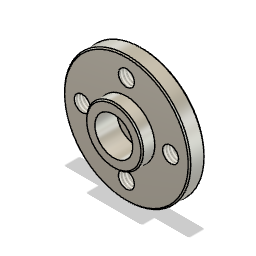
GooGoo (Autodesk Fusion 360 archive; units mm, degrees)
design "Servo Disc"
Autodesk Fusion 360 part; units mm, degrees
note: some values were not read from the file. Set by a fixed rule: which face or edge a step refers to.
sketch "Sketch1" plane through (0, 0, 0) normal (0, 0, 1) x (1, 0, 0)
  circle A0 centre (0, 0) radius 10
  dimension "d1" = 20
  constraint coincident A0.centre origin
  measures "d1" diameter of A0
extrude "Extrude1" add sketch "Sketch1" along normal blind 2.5
sketch "Sketch2" plane through (0, 0, 2.5) normal (0, 0, 1) x (1, 0, 0)
  circle A0 centre (0, 0) radius 10
  circle A1 centre (0, 0) radius 4.5
  dimension "d4" = 9
  constraint concentric A0 A1
  measures "d4" diameter of A1
extrude "Extrude2" add sketch "Sketch2" along normal blind 2 contours A1
sketch "Sketch3" plane through (0, 0, 2.5) normal (0, 0, 1) x (1, 0, 0)
  circle A0 centre (0, 0) radius 4.5
  circle A1 centre (0, 0) radius 10
  line L0 (0, 0) -> (0, 7)
  point P0 (0, 7)
  dimension "d8" = 7
  constraint coincident A0.centre A1.centre
  constraint vertical L0
  constraint coincident P0 L0.end
  measures "d8" distance of A0.centre P0
hole "Hole1" at (0, 7, 2.5) direction (0, 0, -1) diameter 2.529 depth 9 tip angle 118
thread "Thread1" "ISO Metric profile 3.0 M3x0.5 6H"
pattern_circular "C-Pattern1" count 4 over 360 about axis through (0, 0, 0) along (0, 0, 1) of "Hole1"
sketch "Sketch4" plane through (0, 0, 4.5) normal (0, 0, 1) x (1, 0, 0)
  circle A0 centre (0, 0) radius 3
  circle A1 centre (0, 0) radius 4.5
  dimension "d14" = 6
  measures "d14" diameter of A0
extrude "Extrude3" cut sketch "Sketch4" against normal blind 3.5 contours A0
sketch "Sketch5" plane through (0, 0, 1) normal (0, 0, 1) x (1, 0, 0)
  circle A0 centre (0, 0) radius 3
  circle A1 centre (0, 0) radius 1.5
  dimension "d17" = 3
  constraint coincident A0.centre A1.centre
  measures "d17" diameter of A1
extrude "Extrude4" cut sketch "Sketch5" against normal blind 3 contours A1
chamfer "Chamfer1" distance 0.2 angle 45 4 edges at (-4.1955, -1.6273, 4.5) (-9.3233, -3.6162, 2.5) (-9.3233, -3.6162, 0) (-1.3985, -0.5424, 0)

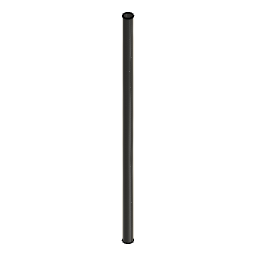
design "20x18x500CR"
Autodesk Fusion 360 part; units mm, degrees
sketch "Sketch1" plane through (0, 0, 0) normal (0, 0, 1) x (1, 0, 0)
  circle A0 centre (0, 0) radius 10
  circle A1 centre (0, 0) radius 9
  dimension "d1" = 20
  dimension "d2" = 18
  constraint coincident A0.centre A1.centre
  measures "d1" diameter of A0
  measures "d2" diameter of A1
extrude "Extrude1" add sketch "Sketch1" along normal blind 500

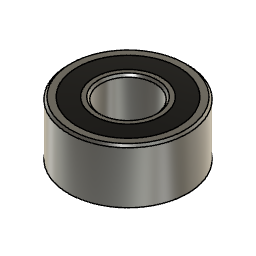
design "5x11x5mmBearing"
Autodesk Fusion 360 part; units mm, degrees
sketch "Sketch1" plane through (0, 0, 0) normal (0, 0, 1) x (1, 0, 0)
  circle A0 centre (0, 0) radius 2.5
  circle A1 centre (0, 0) radius 3.1
  circle A2 centre (0, 0) radius 5.5
  circle A3 centre (0, 0) radius 4.7
  dimension "d1" = 5
  dimension "d2" = 0.6
  dimension "d3" = 11
  dimension "d4" = -0.8
  constraint coincident A0.centre A1.centre
  measures "d1" diameter of A0
  measures "d3" diameter of A2
extrude "Extrude1" add sketch "Sketch1" along normal blind 5 makes body 1 at (5.4932, -0.2742, 3.3333) makes body 2 at (3.0961, -0.1545, 3.3333)
extrude "Extrude2" add sketch "Sketch1" along normal blind 5 separate body contours A3 makes body 3
chamfer "Chamfer1" distance 0.2 angle 45 2 edges at (-5.1278, -1.9889, 5) (-2.3308, 0.904, 5) on bodies 1 2

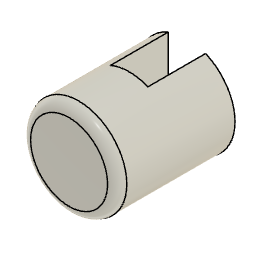
design "PegCR"
Autodesk Fusion 360 part; units mm, degrees
sketch "Sketch1" plane through (0, 0, 0) normal (0, 1, 0) x (1, 0, 0)
  circle A0 centre (0, 0) radius 4
  line L0 (1.55, -6.2) -> (-1.55, -6.2)
  line L1 (-1.55, -6.2) -> (-1.55, 6.2)
  line L2 (-1.55, 6.2) -> (1.55, 6.2)
  line L3 (1.55, 6.2) -> (1.55, -6.2)
  line L4 (1.55, -6.2) -> (-1.55, 6.2) construction
  line L5 (-1.55, -6.2) -> (1.55, 6.2) construction
  dimension "d1" = 8
  dimension "d2" = 3.1
  constraint coincident A0.centre origin
  constraint horizontal L0
  constraint perpendicular L0 L1
  constraint parallel L0 L2
  constraint parallel L1 L3
  constraint coincident L4 A0.centre
  constraint coincident L5 A0.centre
  measures "d1" diameter of A0
  measures "d2" distance of L1.end L2.end
extrude "Extrude1" add sketch "Sketch1" against normal blind 5 contours A0 L3 | A0 L1 L3 | A0 L1
extrude "Extrude2" add sketch "Sketch1" along normal blind 4.8 contours A0 L3 | A0 L1
fillet "Fillet1" radius 0.8 1 edges at (-3.7293, -5, -1.4465)

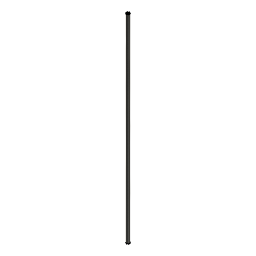
design "8x4x500CR"
Autodesk Fusion 360 part; units mm, degrees
sketch "Sketch1" plane through (0, 0, 0) normal (0, 0, 1) x (1, 0, 0)
  circle A0 centre (0, 0) radius 4
  circle A1 centre (0, 0) radius 2
  dimension "d1" = 8
  dimension "d2" = 4
  constraint coincident A0.centre A1.centre
  measures "d1" diameter of A0
  measures "d2" diameter of A1
extrude "Extrude1" add sketch "Sketch1" along normal blind 500

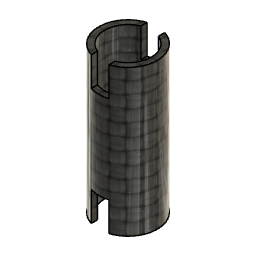
design "10x8x25CR"
Autodesk Fusion 360 part; units mm, degrees
sketch "Sketch1" plane through (0, 0, 0) normal (0, 0, 1) x (1, 0, 0)
  circle A0 centre (0, 0) radius 5
  circle A1 centre (0, 0) radius 4
  line L0 (1.5, 6) -> (-1.5, 6)
  line L1 (-1.5, 6) -> (-1.5, -6)
  line L2 (-1.5, -6) -> (1.5, -6)
  line L3 (1.5, -6) -> (1.5, 6)
  line L4 (1.5, 6) -> (-1.5, -6) construction
  line L5 (-1.5, 6) -> (1.5, -6) construction
  dimension "d1" = 10
  dimension "d2" = 8
  dimension "d3" = 3
  dimension "d4" = 12
  constraint coincident A0.centre A1.centre
  constraint horizontal L0
  constraint perpendicular L0 L1
  constraint parallel L0 L2
  constraint parallel L1 L3
  constraint coincident L4 A0.centre
  constraint coincident L5 A0.centre
  measures "d1" diameter of A0
  measures "d2" diameter of A1
  measures "d3" distance of L1.end L2.end
  measures "d4" distance of L0.end L1.end
extrude "Extrude1" add sketch "Sketch1" along normal blind 25 contours A0 A1 L3 | A0 A1 L1 L3 | A0 A1 L1 L3 | A0 A1 L1
sketch "Sketch2" plane through (0, 0, 25) normal (0, 0, 1) x (-1, 0, 0)
  circle A0 centre (0, 0) radius 4
  circle A1 centre (0, 0) radius 5
  line L0 (-1.5, -6) -> (1.5, -6)
  line L1 (1.5, -6) -> (1.5, 6)
  line L2 (1.5, 6) -> (-1.5, 6)
  line L3 (-1.5, 6) -> (-1.5, -6)
  line L4 (-1.5, -6) -> (1.5, 6) construction
  line L5 (1.5, -6) -> (-1.5, 6) construction
  dimension "d7" = 3
  dimension "d8" = 12
  constraint horizontal L0
  constraint perpendicular L0 L1
  constraint parallel L0 L2
  constraint parallel L1 L3
  constraint coincident L4 A0.centre
  constraint coincident L5 A0.centre
  constraint coincident A0.centre A1.centre
  measures "d7" distance of L1.end L2.end
  measures "d8" distance of L0.end L1.end
extrude "Extrude2" cut sketch "Sketch2" against normal blind 5 contours A0 A1 L1 L3 | A0 A1 L1 L3
extrude "Extrude3" cut sketch "Sketch1" along normal blind 5 contours A0 A1 L1 L3 | A0 A1 L1 L3

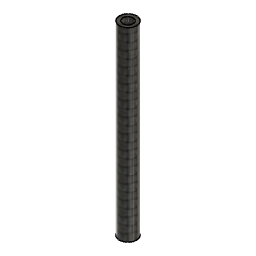
design "5x3x54CR"
Autodesk Fusion 360 part; units mm, degrees
sketch "Sketch1" plane through (0, 0, 0) normal (0, 0, 1) x (1, 0, 0)
  circle A0 centre (0, 0) radius 2.5
  circle A1 centre (0, 0) radius 1.5
  dimension "d1" = 5
  dimension "d2" = 3
  constraint coincident A0.centre A1.centre
  constraint concentric A0 A1
  measures "d1" diameter of A0
  measures "d2" diameter of A1
extrude "Extrude1" add sketch "Sketch1" along normal blind 54

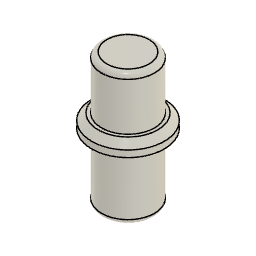
design "BearingCoupler"
Autodesk Fusion 360 part; units mm, degrees
sketch "Sketch1" plane through (0, 0, 0) normal (0, 0, 1) x (1, 0, 0)
  circle A0 centre (0, 0) radius 4
  circle A1 centre (0, 0) radius 5.5
  dimension "d1" = 8
  dimension "d13" = 11
  constraint coincident A0.centre A1.centre
  measures "d1" diameter of A0
  measures "d13" diameter of A1
extrude "Extrude1" add sketch "Sketch1" along normal blind 8 contours A0 makes body 1
extrude "Extrude2" add sketch "Sketch1" against normal blind 2 separate body makes body 2
extrude "Extrude3" add sketch "Sketch1" against normal blind 12 contours A0 bodies 1 2
fillet "Fillet1" radius 0.8 2 edges at (-3.7293, 1.4465, -12) (-3.7293, -1.4465, 8) on bodies 1
chamfer "Chamfer1" distance 1 angle 45 1 edges at (-5.1278, -1.9889, 0) on bodies 1

design "PropStructMount2"
Autodesk Fusion 360 part; units mm, degrees
sketch "Sketch1" plane through (0, 0, 0) normal (0, 1, 0) x (1, 0, 0)
  line L0 (0, 0) -> (-48, 0) construction
  line L1 (-48, 0) -> (-48, -15) construction
  line L2 (-48, -15) -> (-80, -15) construction
  line L3 (0, 0) -> (0, -70) construction
  circle A0 centre (0, -70) radius 10
  circle A1 centre (-80, -15) radius 4
  circle A2 centre (0, -70) radius 14
  circle A3 centre (-80, -15) radius 8
  line L4 (-84.931, -21.2996) -> (-8.6292, -81.0243)
  line L5 (-82.4655, -18.1498) -> (-6.1637, -77.8745)
  line L6 (0, -84) -> (0, -56)
  circle A4 centre (-48, 0) radius 11
  circle A5 centre (-48, 0) radius 15
  line L7 (0, -56) -> (-34.8639, 7.2417)
  line L8 (-2.6272, -57.4483) -> (-37.4911, 5.7933)
  line L9 (-84.7629, -8.5724) -> (-56.9305, 12.0518)
  line L10 (-82.3815, -11.7862) -> (-54.5491, 8.838)
  line L11 (-48, 15) -> (0, 15)
  line L12 (0, 15) -> (0, -56)
  dimension "d1" = 48
  dimension "d2" = 15
  dimension "d3" = 32
  dimension "d4" = 70
  dimension "d5" = 20
  dimension "d6" = 8
  dimension "d7" = 4
  dimension "d8" = 4
  dimension "d9" = 22
  dimension "d10" = 4
  dimension "d11" = -3
  dimension "d12" = 48
  constraint coincident L0.start L3.start
  constraint horizontal L0
  constraint perpendicular L0 L1
  constraint perpendicular L1 L2
  constraint perpendicular L0 L3
  constraint coincident L3.end A0.centre
  constraint coincident L2.end A1.centre
  constraint coincident A3 L4.start
  constraint coincident A2 L4.end
  constraint tangent A2 L4
  constraint coincident A1 L5.start
  constraint coincident A0 L5.end
  constraint tangent A0 L5
  constraint tangent A3 L4
  constraint tangent A1 L5
  constraint coincident A2 L6.start
  constraint coincident L3 L6.end
  constraint coincident A2 L6.end
  constraint parallel L3 L6
  constraint coincident L0.end L1.start
  constraint coincident A5 L7.end
  constraint tangent A5 L7
  constraint coincident A3 L9.start
  constraint coincident A5 L9.end
  constraint coincident A1 L10.start
  constraint coincident A4 L10.end
  constraint tangent A4 L10
  constraint tangent A5 L9
  constraint tangent A3 L9
  constraint tangent A1 L10
  constraint coincident A5 L11.start
  constraint parallel L0 L11
  constraint perpendicular L11 L12
  measures "d1" distance of L0.start L0.end
  measures "d2" distance of L0.end L1.end
  measures "d3" distance of L1.end L2.end
  measures "d4" distance of L0.start L3.end
  measures "d5" diameter of A0
  measures "d6" diameter of A1
  measures "d8" distance of A1
  measures "d9" diameter of A4
  measures "d12" distance of L11.start L11.end
extrude "Extrude1" add sketch "Sketch1" along normal blind 10 contours A0 A2 L5 L6 | A0 A2 L5 L6 | A2 A5 L7 L8 | A5 L7 L11 L12 | A2 A3 L5 A5 L8 L10 | A2 A3 L4 L5 | A5 | A1 A3 L5 L10 | A1 A3 L5 L10 | A3 A5 L9 L10
sketch "Sketch2" plane through (0, 0, 0) normal (0, -1, 0) x (1, 0, 0)
  circle A0 centre (-48, 0) radius 11
  circle A1 centre (-80, 15) radius 4
  arc A2 (-56.9305, -12.0518) -> (-48, -15) centre (-48, 0) ccw
  line L0 (-48, -15) -> (0, -15)
  line L1 (0, -15) -> (0, 60)
  arc A3 (0, 80) -> (0, 60) centre (0, 70) ccw
  line L2 (0, 80) -> (0, 84)
  arc A4 (0, 84) -> (-8.6292, 81.0243) centre (0, 70) ccw
  line L3 (-8.6292, 81.0243) -> (-84.931, 21.2996)
  arc A5 (-84.931, 21.2996) -> (-84.7629, 8.5724) centre (-80, 15) ccw
  line L4 (-84.7629, 8.5724) -> (-56.9305, -12.0518)
  circle A6 centre (-48, 0) radius 15
  circle A7 centre (-80, 15) radius 8
  circle A8 centre (0, 70) radius 14
  line L5 (-78.1065, 22.7727) -> (-44.4498, 14.5738)
  line L6 (-82.4655, 18.1498) -> (-6.1637, 77.8745)
  line L7 (0, 56) -> (-34.8639, -7.2417)
  circle A9 centre (0, 70) radius 10
  line L8 (-78.8166, 19.8579) -> (-45.1598, 11.659)
  line L9 (-82.3815, 11.7862) -> (-54.5491, -8.838)
  line L10 (-3.503, 57.9311) -> (-38.3668, -5.3106)
  line L11 (-13.8792, 71.8353) -> (-33.4434, 3.6203)
  line L12 (-16.7629, 72.6624) -> (-36.3272, 4.4473)
  circle A10 centre (0, -15) radius 34.2773
  circle A11 centre (0, -15) radius 38.2773
  dimension "d17" = 3
  dimension "d18" = -4
  dimension "d19" = 4
  dimension "d21" = 3
  dimension "d22" = 4
  constraint concentric A0 A6
  constraint concentric A1 A7
  constraint concentric A3 A8
  constraint coincident L2.end A8
  constraint coincident A7 L5.start
  constraint coincident A6 L5.end
  constraint tangent A6 L5
  constraint tangent A7 L5
  constraint coincident A1 L6.start
  constraint coincident A3 L6.end
  constraint tangent A3 L6
  constraint tangent A1 L6
  constraint coincident A8 L7.start
  constraint coincident L1 L7.start
  constraint coincident A6 L7.end
  constraint tangent A6 L7
  constraint concentric A8 A9
  constraint coincident L1.end A9
  constraint coincident A8 L11.start
  constraint coincident L6 L11.start
  constraint coincident A6 L11.end
  constraint coincident L10 L11.end
  constraint coincident L0.end L1.start
  constraint tangent L7 A10
extrude "Extrude2" cut sketch "Sketch2" against normal through all contours A8 L10 L11 | A6 A7 L8 L9 | A6 L5 L6 L12 | L1 L7 A11 | L0 A6 A11 | L0 A6 L7 A10 A11 | L0 L1 A10 picked at (-19.1897, -2.6862)
fillet "Fillet1" radius 1.5 2 edges at (-13.8792, 5, 71.8353) (-33.4434, 5, 3.6203)
fillet "Fillet2" radius 2 2 edges at (-17.9036, 5, 68.6853) (-76.9267, 5, 22.4853)
fillet "Fillet3" radius 2 1 edges at (-35.3093, 5, 7.9966)
fillet "Fillet4" radius 2 4 edges at (-53.9041, 5, 13.7892) (-72.749, 5, 18.3799) (-76.815, 5, 7.6614) (-62.7427, 5, -2.7664)
mirror "Mirror1" about plane through (0, 0, 0) normal (1, 0, 0) of bodies 1 merged
fillet "Fillet5" radius 1.2 2 edges at (-21.7936, 5, 16.4673) (21.7936, 5, 16.4673)
fillet "Fillet6" radius 3 3 edges at (-4.2103, 5, 56.6481) (0, 5, 56) (4.2103, 5, 56.6481)
ref_plane "WorkPlane1" through (0, 7, 0) normal (0, 1, 0) x (0, 0, 1)
sketch "Sketch3" plane through (0, 7, 0) normal (0, 1, 0) x (1, 0, 0)
  line L0 (0, 0) -> (48, 0) construction
  circle A0 centre (48, 0) radius 11.5
  circle A1 centre (48, 0) radius 7
  line L1 (0, 0) -> (0, -5) construction
  circle A2 centre (-48, 0) radius 7
  circle A3 centre (-48, 0) radius 11.5
  dimension "d36" = 48
  dimension "d37" = 23
  dimension "d38" = 14
  dimension "d39" = 5
  constraint coincident L0.start L1.start
  constraint horizontal L0
  constraint coincident L0.end A0.centre
  constraint concentric A0 A1
  constraint perpendicular L0 L1
  constraint symmetric A0 L1 A3
  constraint symmetric A1 L1 A2
  measures "d36" distance of L0.start L0.end
  measures "d37" diameter of A0
  measures "d38" diameter of A1
  measures "d39" distance of L0.start L1.end
extrude "Extrude3" add sketch "Sketch3" along normal blind 3
fillet "Fillet7" radius 1.5 48 faces at (19.0968, 3.3333, 18.765) (8.2897, 3.3333, 40.9627) (0, 3.3333, 52.786) (-8.2897, 3.3333, 40.9627) (-19.6699, 3.3333, 19.3747) (-11.4237, 6.6667, 21.5329) (20.521, 3.3333, 48.6773) (28.8377, 3.3333, 14.5841) (12.8668, 3.3333, 40.9455) (5.4179, 3.3333, 55.2754) (10.3943, 6.6667, 60.6213) (13.7109, 3.3333, 65.7014) (-12.8668, 6.6667, 40.9455) (-5.4179, 3.3333, 55.2754) (-10.3943, 6.6667, 60.6213) (-13.7109, 3.3333, 65.7014) (-20.521, 3.3333, 48.6773) (-28.8377, 3.3333, 14.5841) (63.4298, 3.3333, 19.1974) (73.7897, 6.6667, 21.9706) (56.7056, 3.3333, 38.3132) (22.5975, 3.3333, 64.9988) (24.4878, 3.3333, 45.7279) (37.4225, 6.6667, 10.6509) (38.056, 3.3333, 11.2302) (-63.4298, 3.3333, 19.1974) (-73.7897, 6.6667, 21.9706) (-56.7056, 6.6667, 38.3132) (-22.5975, 3.3333, 64.9988) (-24.4878, 3.3333, 45.7279) (-37.4225, 6.6667, 10.6509) (-38.056, 3.3333, 11.2302) (-61.0351, 6.6667, 7.4219) (-64.8968, 3.3333, -0.6439) (-71.7184, 6.6667, 3.8847) (-75.1274, 3.3333, 6.7064) (-72.0454, 6.6667, 14.1488) (-71.4826, 6.6667, 17.0228) (-65.8711, 3.3333, 16.7044) (-58.3295, 3.3333, 14.8574) (71.7184, 6.6667, 3.8847) (64.8968, 3.3333, -0.6439) (61.0351, 6.6667, 7.4219) (58.3295, 3.3333, 14.8574) (65.8711, 3.3333, 16.7044) (71.4826, 6.6667, 17.0228) (72.0454, 6.6667, 14.1488) (75.1274, 3.3333, 6.7064)
fillet "Fillet8" radius 1 24 edges at (46.7801, 0, 51.162) (87.9993, 0, 14.8944) (70.8467, 0, -1.7397) (44.8053, 0, -14.6559) (32.4409, 0, -2.8465) (0, 0, 19.2773) (-32.4409, 0, -2.8465) (-44.8053, 0, -14.6559) (-70.8467, 0, -1.7397) (-87.9993, 0, 14.8944) (-46.7801, 0, 51.162) (0, 0, 84) (46.7801, 10, 51.162) (87.9993, 10, 14.8944) (70.8467, 10, -1.7397) (44.8053, 10, -14.6559) (32.4409, 10, -2.8465) (0, 10, 19.2773) (-32.4409, 10, -2.8465) (-44.8053, 10, -14.6559) (-70.8467, 10, -1.7397) (-87.9993, 10, 14.8944) (-46.7801, 10, 51.162) (0, 10, 84)
sketch "Sketch5" plane through (0, 0, 0) normal (0, -1, 0) x (1, 0, 0)
  arc A0 (-69.1932, 19.0575) -> (-73.514, 15.427) centre (-70.0216, 15.657) ccw
  line L0 (-69.1932, 19.0575) -> (-73.2748, 20.0518)
  arc A1 (-74.6037, 26.2084) -> (-73.2748, 20.0518) centre (-72.4464, 23.4524) ccw
  line L1 (-74.6037, 26.2084) -> (-23.6831, 66.0662)
  arc A2 (-18.1614, 62.3452) -> (-23.6831, 66.0662) centre (-21.5258, 63.3101) ccw
  line L2 (-18.1614, 62.3452) -> (-17.3357, 65.2243)
  arc A3 (-11.6548, 65.4817) -> (-17.3357, 65.2243) centre (-14.452, 64.3973) ccw
  arc A4 (-11.6548, 65.4817) -> (-6.1894, 59.1399) centre (0, 70) ccw
  arc A5 (-4.4767, 53.0578) -> (-6.1894, 59.1399) centre (-8.4176, 55.2303) ccw
  line L3 (-4.4767, 53.0578) -> (-25.7061, 14.5485)
  arc A6 (-31.2171, 16.8239) -> (-25.7061, 14.5485) centre (-28.3333, 15.9968) ccw
  line L4 (-31.2171, 16.8239) -> (-32.8149, 11.2527)
  arc A7 (-38.613, 9.7022) -> (-32.8149, 11.2527) centre (-36.1793, 12.2176) ccw
  arc A8 (-38.613, 9.7022) -> (-44.8048, 13.1164) centre (-48, 0) ccw
  line L5 (-44.8048, 13.1164) -> (-58.1619, 16.3703)
  arc A9 (-56.7276, 10.2995) -> (-58.1619, 16.3703) centre (-58.9903, 12.9697) ccw
  arc A10 (-56.7276, 10.2995) -> (-61.457, 1.0764) centre (-48, 0) ccw
  arc A11 (-67.0297, -1.4566) -> (-61.457, 1.0764) centre (-64.9459, 1.3555) ccw
  line L6 (-67.0297, -1.4566) -> (-75.4023, 4.7476)
  arc A12 (-75.6571, 10.1638) -> (-75.4023, 4.7476) centre (-73.3185, 7.5597) ccw
  arc A13 (-75.6571, 10.1638) -> (-73.514, 15.427) centre (-80, 15) ccw
  arc A14 (17.2942, 17.4574) -> (20.9284, 21.1437) centre (18.5639, 19.8402) ccw
  arc A15 (17.2942, 17.4574) -> (-17.2942, 17.4574) centre (0, -15) ccw
  arc A16 (-20.9284, 21.1437) -> (-17.2942, 17.4574) centre (-18.5639, 19.8402) ccw
  line L7 (-20.9284, 21.1437) -> (-3.9408, 51.9585)
  arc A17 (3.9408, 51.9585) -> (-3.9408, 51.9585) centre (0, 49.786) ccw
  line L8 (3.9408, 51.9585) -> (20.9284, 21.1437)
  circle A18 centre (0, 70) radius 10
  circle A19 centre (48, 0) radius 11
  circle A20 centre (80, 15) radius 4
  circle A21 centre (-80, 15) radius 4
  circle A22 centre (-48, 0) radius 11
  arc A23 (73.514, 15.427) -> (69.1932, 19.0575) centre (70.0216, 15.657) ccw
  arc A24 (73.514, 15.427) -> (75.6571, 10.1638) centre (80, 15) ccw
  arc A25 (75.4023, 4.7476) -> (75.6571, 10.1638) centre (73.3185, 7.5597) ccw
  line L9 (75.4023, 4.7476) -> (67.0297, -1.4566)
  arc A26 (61.457, 1.0764) -> (67.0297, -1.4566) centre (64.9459, 1.3555) ccw
  arc A27 (61.457, 1.0764) -> (56.7276, 10.2995) centre (48, 0) ccw
  arc A28 (58.1619, 16.3703) -> (56.7276, 10.2995) centre (58.9903, 12.9697) ccw
  line L10 (58.1619, 16.3703) -> (44.8048, 13.1164)
  arc A29 (44.8048, 13.1164) -> (38.613, 9.7022) centre (48, 0) ccw
  arc A30 (32.8149, 11.2527) -> (38.613, 9.7022) centre (36.1793, 12.2176) ccw
  line L11 (32.8149, 11.2527) -> (31.2171, 16.8239)
  arc A31 (25.7061, 14.5485) -> (31.2171, 16.8239) centre (28.3333, 15.9968) ccw
  line L12 (25.7061, 14.5485) -> (4.4767, 53.0578)
  arc A32 (6.1894, 59.1399) -> (4.4767, 53.0578) centre (8.4176, 55.2303) ccw
  arc A33 (6.1894, 59.1399) -> (11.6548, 65.4817) centre (0, 70) ccw
  arc A34 (17.3357, 65.2243) -> (11.6548, 65.4817) centre (14.452, 64.3973) ccw
  line L13 (17.3357, 65.2243) -> (18.1614, 62.3452)
  arc A35 (23.6831, 66.0662) -> (18.1614, 62.3452) centre (21.5258, 63.3101) ccw
  line L14 (23.6831, 66.0662) -> (74.6037, 26.2084)
  arc A36 (73.2748, 20.0518) -> (74.6037, 26.2084) centre (72.4464, 23.4524) ccw
  line L15 (73.2748, 20.0518) -> (69.1932, 19.0575)
  line L16 (84.3146, 20.5122) -> (8.0129, 80.2369)
  arc A37 (8.0129, 80.2369) -> (-8.0129, 80.2369) centre (0, 70) ccw
  line L17 (-8.0129, 80.2369) -> (-84.3146, 20.5122)
  arc A38 (-84.3146, 20.5122) -> (-84.1676, 9.3758) centre (-80, 15) ccw
  line L18 (-84.1676, 9.3758) -> (-56.3352, -11.2483)
  arc A39 (-56.3352, -11.2483) -> (-35.7396, -6.7589) centre (-48, 0) ccw
  line L19 (-35.7396, -6.7589) -> (-30.8937, 2.0314)
  arc A40 (30.8937, 2.0314) -> (-30.8937, 2.0314) centre (0, -15) ccw
  line L20 (30.8937, 2.0314) -> (35.7396, -6.7589)
  arc A41 (35.7396, -6.7589) -> (56.3352, -11.2483) centre (48, 0) ccw
  line L21 (56.3352, -11.2483) -> (84.1676, 9.3758)
  arc A42 (84.1676, 9.3758) -> (84.3146, 20.5122) centre (80, 15) ccw
  circle A43 centre (-48, 0) radius 11.1
  circle A44 centre (48, 0) radius 11.1
  dimension "d55" = 22.2
  dimension "d56" = 22.2
  constraint concentric A8 A43
  constraint concentric A19 A44
  measures "d55" diameter of A43
  measures "d56" diameter of A44
extrude "Extrude5" cut sketch "Sketch5" against normal blind 7 contours A43 | A44
fillet "Fillet9" radius 1 2 edges at (-58.3488, 0, 4.0139) (37.6512, 0, 4.0139)
chamfer "Chamfer1" distance 1 angle 45 2 edges at (41.4737, 7, -2.5313) (-54.5263, 7, -2.5313)
sketch "Sketch4" plane through (0, 0, 0) normal (0, -1, 0) x (1, 0, 0)
  arc A0 (-69.1932, 19.0575) -> (-73.514, 15.427) centre (-70.0216, 15.657) ccw
  line L0 (-69.1932, 19.0575) -> (-73.2748, 20.0518)
  arc A1 (-74.6037, 26.2084) -> (-73.2748, 20.0518) centre (-72.4464, 23.4524) ccw
  line L1 (-74.6037, 26.2084) -> (-23.6831, 66.0662)
  arc A2 (-18.1614, 62.3452) -> (-23.6831, 66.0662) centre (-21.5258, 63.3101) ccw
  line L2 (-18.1614, 62.3452) -> (-17.3357, 65.2243)
  arc A3 (-11.6548, 65.4817) -> (-17.3357, 65.2243) centre (-14.452, 64.3973) ccw
  arc A4 (-11.6548, 65.4817) -> (-6.1894, 59.1399) centre (0, 70) ccw
  arc A5 (-4.4767, 53.0578) -> (-6.1894, 59.1399) centre (-8.4176, 55.2303) ccw
  line L3 (-4.4767, 53.0578) -> (-25.7061, 14.5485)
  arc A6 (-31.2171, 16.8239) -> (-25.7061, 14.5485) centre (-28.3333, 15.9968) ccw
  line L4 (-31.2171, 16.8239) -> (-32.8149, 11.2527)
  arc A7 (-38.613, 9.7022) -> (-32.8149, 11.2527) centre (-36.1793, 12.2176) ccw
  arc A8 (-38.613, 9.7022) -> (-44.8048, 13.1164) centre (-48, 0) ccw
  line L5 (-44.8048, 13.1164) -> (-58.1619, 16.3703)
  arc A9 (-56.7276, 10.2995) -> (-58.1619, 16.3703) centre (-58.9903, 12.9697) ccw
  arc A10 (-56.7276, 10.2995) -> (-61.457, 1.0764) centre (-48, 0) ccw
  arc A11 (-67.0297, -1.4566) -> (-61.457, 1.0764) centre (-64.9459, 1.3555) ccw
  line L6 (-67.0297, -1.4566) -> (-75.4023, 4.7476)
  arc A12 (-75.6571, 10.1638) -> (-75.4023, 4.7476) centre (-73.3185, 7.5597) ccw
  arc A13 (-75.6571, 10.1638) -> (-73.514, 15.427) centre (-80, 15) ccw
  arc A14 (17.2942, 17.4574) -> (20.9284, 21.1437) centre (18.5639, 19.8402) ccw
  arc A15 (17.2942, 17.4574) -> (-17.2942, 17.4574) centre (0, -15) ccw
  arc A16 (-20.9284, 21.1437) -> (-17.2942, 17.4574) centre (-18.5639, 19.8402) ccw
  line L7 (-20.9284, 21.1437) -> (-3.9408, 51.9585)
  arc A17 (3.9408, 51.9585) -> (-3.9408, 51.9585) centre (0, 49.786) ccw
  line L8 (3.9408, 51.9585) -> (20.9284, 21.1437)
  circle A18 centre (0, 70) radius 10
  circle A19 centre (80, 15) radius 4
  circle A20 centre (-80, 15) radius 4
  arc A21 (73.514, 15.427) -> (69.1932, 19.0575) centre (70.0216, 15.657) ccw
  arc A22 (73.514, 15.427) -> (75.6571, 10.1638) centre (80, 15) ccw
  arc A23 (75.4023, 4.7476) -> (75.6571, 10.1638) centre (73.3185, 7.5597) ccw
  line L9 (75.4023, 4.7476) -> (67.0297, -1.4566)
  arc A24 (61.457, 1.0764) -> (67.0297, -1.4566) centre (64.9459, 1.3555) ccw
  arc A25 (61.457, 1.0764) -> (56.7276, 10.2995) centre (48, 0) ccw
  arc A26 (58.1619, 16.3703) -> (56.7276, 10.2995) centre (58.9903, 12.9697) ccw
  line L10 (58.1619, 16.3703) -> (44.8048, 13.1164)
  arc A27 (44.8048, 13.1164) -> (38.613, 9.7022) centre (48, 0) ccw
  arc A28 (32.8149, 11.2527) -> (38.613, 9.7022) centre (36.1793, 12.2176) ccw
  line L11 (32.8149, 11.2527) -> (31.2171, 16.8239)
  arc A29 (25.7061, 14.5485) -> (31.2171, 16.8239) centre (28.3333, 15.9968) ccw
  line L12 (25.7061, 14.5485) -> (4.4767, 53.0578)
  arc A30 (6.1894, 59.1399) -> (4.4767, 53.0578) centre (8.4176, 55.2303) ccw
  arc A31 (6.1894, 59.1399) -> (11.6548, 65.4817) centre (0, 70) ccw
  arc A32 (17.3357, 65.2243) -> (11.6548, 65.4817) centre (14.452, 64.3973) ccw
  line L13 (17.3357, 65.2243) -> (18.1614, 62.3452)
  arc A33 (23.6831, 66.0662) -> (18.1614, 62.3452) centre (21.5258, 63.3101) ccw
  line L14 (23.6831, 66.0662) -> (74.6037, 26.2084)
  arc A34 (73.2748, 20.0518) -> (74.6037, 26.2084) centre (72.4464, 23.4524) ccw
  line L15 (73.2748, 20.0518) -> (69.1932, 19.0575)
  line L16 (84.3146, 20.5122) -> (8.0129, 80.2369)
  arc A35 (8.0129, 80.2369) -> (-8.0129, 80.2369) centre (0, 70) ccw
  line L17 (-8.0129, 80.2369) -> (-84.3146, 20.5122)
  arc A36 (-84.3146, 20.5122) -> (-84.1676, 9.3758) centre (-80, 15) ccw
  line L18 (-84.1676, 9.3758) -> (-56.3352, -11.2483)
  arc A37 (-56.3352, -11.2483) -> (-35.7396, -6.7589) centre (-48, 0) ccw
  line L19 (-35.7396, -6.7589) -> (-30.8937, 2.0314)
  arc A38 (30.8937, 2.0314) -> (-30.8937, 2.0314) centre (0, -15) ccw
  line L20 (30.8937, 2.0314) -> (35.7396, -6.7589)
  arc A39 (35.7396, -6.7589) -> (56.3352, -11.2483) centre (48, 0) ccw
  line L21 (56.3352, -11.2483) -> (84.1676, 9.3758)
  arc A40 (84.1676, 9.3758) -> (84.3146, 20.5122) centre (80, 15) ccw
  circle A41 centre (0, 70) radius 10.1
  circle A42 centre (-80, 15) radius 4.2
  circle A43 centre (80, 15) radius 4.2
  circle A44 centre (-48, 0) radius 12.1
  circle A45 centre (48, 0) radius 12.1
  dimension "d49" = 20.2
  dimension "d50" = 8.4
  dimension "d51" = 8.4
  constraint concentric A4 A41
  constraint concentric A13 A42
  constraint concentric A19 A43
  measures "d49" diameter of A41
  measures "d50" diameter of A42
  measures "d51" diameter of A43
extrude "Extrude4" cut sketch "Sketch4" against normal blind 10 contours A41 | A42 | A43
chamfer "Chamfer2" distance 0.7 angle 45 3 faces at (10.0874, 6.6667, 69.4966) (84.1948, 6.6667, 14.7906) (-75.8052, 6.6667, 14.7906)
chamfer "Chamfer3" distance 0.7 angle 45 2 edges at (41.4737, 10, -2.5313) (-54.5263, 10, -2.5313)

design "10x8x22CR"
Autodesk Fusion 360 part; units mm, degrees
sketch "Sketch1" plane through (0, 0, 0) normal (0, 0, 1) x (1, 0, 0)
  circle A0 centre (0, 0) radius 5
  circle A1 centre (0, 0) radius 4
  line L0 (1.5, 6) -> (-1.5, 6)
  line L1 (-1.5, 6) -> (-1.5, -6)
  line L2 (-1.5, -6) -> (1.5, -6)
  line L3 (1.5, -6) -> (1.5, 6)
  line L4 (1.5, 6) -> (-1.5, -6) construction
  line L5 (-1.5, 6) -> (1.5, -6) construction
  dimension "d1" = 10
  dimension "d2" = 8
  dimension "d3" = 3
  dimension "d4" = 12
  constraint coincident A0.centre A1.centre
  constraint concentric A0 A1
  constraint horizontal L0
  constraint perpendicular L0 L1
  constraint parallel L0 L2
  constraint parallel L1 L3
  constraint coincident L4 A0.centre
  constraint coincident L5 A0.centre
  measures "d1" diameter of A0
  measures "d2" diameter of A1
  measures "d3" distance of L1.end L2.end
  measures "d4" distance of L0.end L1.end
extrude "Extrude1" add sketch "Sketch1" along normal blind 22 contours A0 A1 L3 | A0 A1 L1 L3 | A0 A1 L1 L3 | A0 A1 L1
extrude "Extrude2" cut sketch "Sketch1" along normal blind 5 contours A0 A1 L1 L3 | A0 A1 L1 L3
sketch "Sketch2" plane through (0, 0, 22) normal (0, 0, 1) x (-1, 0, 0)
  circle A0 centre (0, 0) radius 4
  circle A1 centre (0, 0) radius 5
  line L0 (6, 2.5) -> (-6, 2.5)
  line L1 (-6, 2.5) -> (-6, -2.5)
  line L2 (-6, -2.5) -> (6, -2.5)
  line L3 (6, -2.5) -> (6, 2.5)
  line L4 (6, 2.5) -> (-6, -2.5) construction
  line L5 (-6, 2.5) -> (6, -2.5) construction
  dimension "d9" = 12
  dimension "d10" = 5
  constraint horizontal L0
  constraint perpendicular L0 L1
  constraint parallel L0 L2
  constraint parallel L1 L3
  constraint coincident L4 A0.centre
  constraint coincident L5 A0.centre
  constraint coincident A0.centre A1.centre
  measures "d9" distance of L1.end L2.end
  measures "d10" distance of L0.end L1.end
extrude "Extrude3" cut sketch "Sketch2" against normal blind 5 contours A0 A1 L0 L2 | A0 A1 L0 L2

design "M2x20"
Autodesk Fusion 360 part; units mm, degrees
cylinder "CylinderPrimitive1" add diameter 3.4 height 1.5 placed x (1, 0, 0) y (0, 1, 0) z (0, 0, 1) at (0, 0, 0)
cylinder "CylinderPrimitive2" add diameter 2 height 20 placed x (1, 0, 0) y (0, 1, 0) z (0, 0, 1) at (0, 0, 1.5)

design "5x3x195.5CR"
Autodesk Fusion 360 part; units mm, degrees
sketch "Sketch1" plane through (0, 0, 0) normal (0, 0, 1) x (1, 0, 0)
  circle A0 centre (0, 0) radius 2.5
  circle A1 centre (0, 0) radius 1.5
  dimension "d1" = 5
  dimension "d2" = 3
  constraint coincident A0.centre A1.centre
  measures "d1" diameter of A0
  measures "d2" diameter of A1
extrude "Extrude1" add sketch "Sketch1" along normal blind 195.5

design "10x8x67CR"
Autodesk Fusion 360 part; units mm, degrees
sketch "Sketch1" plane through (0, 0, 0) normal (0, 0, 1) x (1, 0, 0)
  circle A0 centre (0, 0) radius 5
  circle A1 centre (0, 0) radius 4
  line L0 (1.5, 6) -> (-1.5, 6)
  line L1 (-1.5, 6) -> (-1.5, -6)
  line L2 (-1.5, -6) -> (1.5, -6)
  line L3 (1.5, -6) -> (1.5, 6)
  line L4 (1.5, 6) -> (-1.5, -6) construction
  line L5 (-1.5, 6) -> (1.5, -6) construction
  dimension "d1" = 10
  dimension "d2" = 8
  dimension "d3" = 3
  dimension "d4" = 12
  constraint coincident A0.centre A1.centre
  constraint concentric A0 A1
  constraint horizontal L0
  constraint perpendicular L0 L1
  constraint parallel L0 L2
  constraint parallel L1 L3
  constraint coincident L4 A0.centre
  constraint coincident L5 A0.centre
  measures "d1" diameter of A0
  measures "d2" diameter of A1
  measures "d3" distance of L1.end L2.end
  measures "d4" distance of L0.end L1.end
extrude "Extrude1" add sketch "Sketch1" along normal blind 67 contours A0 A1 L3 | A0 A1 L1 L3 | A0 A1 L1 L3 | A0 A1 L1
sketch "Sketch2" plane through (0, 0, 67) normal (0, 0, 1) x (-1, 0, 0)
  circle A0 centre (0, 0) radius 4
  circle A1 centre (0, 0) radius 5
  line L0 (-1.5, -6) -> (1.5, -6)
  line L1 (1.5, -6) -> (1.5, 6)
  line L2 (1.5, 6) -> (-1.5, 6)
  line L3 (-1.5, 6) -> (-1.5, -6)
  line L4 (-1.5, -6) -> (1.5, 6) construction
  line L5 (1.5, -6) -> (-1.5, 6) construction
  dimension "d7" = 3
  dimension "d8" = 12
  constraint horizontal L0
  constraint perpendicular L0 L1
  constraint parallel L0 L2
  constraint parallel L1 L3
  constraint coincident L4 A0.centre
  constraint coincident L5 A0.centre
  constraint coincident A0.centre A1.centre
  measures "d7" distance of L1.end L2.end
  measures "d8" distance of L0.end L1.end
extrude "Extrude2" cut sketch "Sketch2" against normal blind 5 contours A0 A1 L1 L3 | A0 A1 L1 L3
extrude "Extrude3" cut sketch "Sketch1" along normal blind 5 contours A0 A1 L1 L3 | A0 A1 L1 L3
